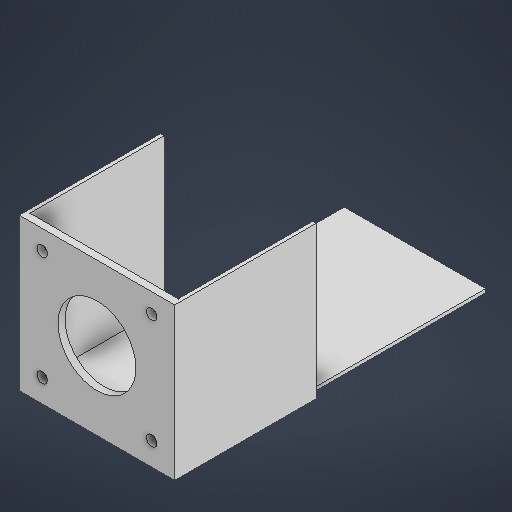
# Autodesk Inventor part: Motor Stand
Saved by Autodesk Inventor 2025.3 (Build 293356030, 356C)
## iProperties
Created: 2025-09-30
Part Number: Motor Stand
Material: Generic
Document SubType Name: Modeling
Designer: yo
Density: 1 g/cm^3
Appearance: Default
Author: yo
Autodesk Inventor part; units mm, degrees
ref_plane "YZ Plane" through (0, 0, 0) normal (1, 0, 0) x (0, 1, 0)
ref_plane "XZ Plane" through (0, 0, 0) normal (0, 1, 0) x (-1, 0, 0)
ref_plane "XY Plane" through (0, 0, 0) normal (0, 0, 1) x (1, 0, 0)
sketch "Sketch1" plane through (0, 0, 0) normal (0, 0, 1) x (1, 0, 0)
  line L0 (-22, 22) -> (22, 22)
  line L1 (22, 22) -> (22, -22)
  line L2 (22, -22) -> (-22, -22)
  line L3 (-22, -22) -> (-22, 22)
  circle A0 centre (15.5, 15.5) radius 1.475
  circle A1 centre (-15.5, 15.5) radius 1.475
  circle A2 centre (15.5, -15.5) radius 1.475
  circle A3 centre (-15.5, -15.5) radius 1.475
  line L4 (-15.5, 15.5) -> (15.5, 15.5) construction
  line L5 (15.5, 15.5) -> (15.5, -15.5) construction
  circle A4 centre (0, 0) radius 11
  line L6 (-21, 21) -> (21, 21)
  line L7 (21, 21) -> (21, -21)
  line L8 (21, -21) -> (-21, -21)
  line L9 (-21, -21) -> (-21, 21)
  line L10 (21, 21) -> (22, 21)
  line L11 (-21, 21) -> (-22, 21)
  point P0 (0, 22)
  point P1 (22, 0)
  point P2 (15.5, 0)
  point P3 (0, 15.5)
  point P4 (0, 21)
  point P5 (21, 0)
  dimension "d0" = 44
  dimension "d1" = 2.95
  dimension "d4" = 31
  dimension "d7" = 31
  dimension "d10" = 22
  dimension "d11" = 42
  constraints: 24 end point, 6 midpoint, 5 centre point, 5 parallel, 5 perpendicular, 4 horizontal, 3 horizontal alignment, 3 point on line, 3 vertical alignment, 1 coincident, 1 vertical, 6 other
  measures "d0" distance of L0.start L0.end
  measures "d1" diameter of A0
  measures "d4" distance of L4.end L4.start
  measures "d7" distance of L4.end L5.end
  measures "d10" diameter of A4
  measures "d11" distance of L7.end L8.end
extrude "Extrusion1" add sketch "Sketch1" along normal blind 2 contours L11 L9 L8 L7 L10 L1 L2 L3 | L6 L7 L8 L9
extrude "Extrusion2" add sketch "Sketch1" against normal blind 38 contours L11 L9 L8 L7 L10 L1 L2 L3
sketch "Sketch2" plane through (0, 0, -38) normal (0, 0, -1) x (-1, 0, 0)
  line L0 (21, -21) -> (21, 21) projected
  line L1 (21, -21) -> (22, -21)
  line L2 (22, 21) -> (22, -22) projected
  line L3 (-21, -21) -> (-21, 21) projected
  line L4 (-21, -21) -> (-22, -21)
  line L5 (-22, 21) -> (-22, -22) projected
  line L6 (21, -21) -> (-21, -21) projected
  line L7 (-22, -22) -> (22, -22) projected
  line L8 (-20, -21) -> (-20, -22)
  line L9 (20, -21) -> (20, -22)
  line L10 (-20, -21.5) -> (20, -21.5) construction
  point P0 (0, 0)
  point P1 (0, -21.5)
  dimension "d16" = 40
  constraints: 10 end point, 7 point on line, 3 midpoint, 2 perpendicular, 1 horizontal, 1 vertical alignment
  measures "d16" distance between parallel lines of L9 L8
extrude "Extrusion3" add sketch "Sketch2" along normal blind 50 contours L9 L7 L8 L6
body "Solid1"
